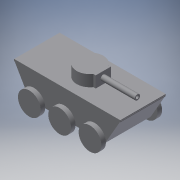
# Autodesk Inventor part: Part1
Saved by Autodesk Inventor 2019 (Build 230136000, 136)
## iProperties
Created: 2019-04-02
Part Number: Part1
Material: Generic
Document SubType Name: Modeling
Designer: Dainis-PC
Density: 1 g/cm^3
Appearance: Default
Author: Dainis-PC
Autodesk Inventor part; units mm, degrees
ref_plane "YZ Plane" through (0, 0, 0) normal (1, 0, 0) x (0, 1, 0)
ref_plane "XZ Plane" through (0, 0, 0) normal (0, 1, 0) x (-1, 0, 0)
ref_plane "XY Plane" through (0, 0, 0) normal (0, 0, 1) x (1, 0, 0)
sketch "Sketch1" plane through (0, 0, 0) normal (0, 0, 1) x (1, 0, 0)
  line L0 (0, 0) -> (200, 0)
  line L1 (0, 0) -> (-40, 69.282)
  line L2 (0, 0) -> (80, 0) construction
  line L3 (200, 0) -> (240, 69.282)
  line L4 (200, 0) -> (280, 0) construction
  line L5 (-40, 69.282) -> (240, 69.282)
  dimension "d0" = 200
  dimension "d1" = 80
  dimension "d2" = 120
  dimension "d3" = 80
  dimension "d4" = 60
  constraints: 12 end point, 3 horizontal, 2 equal length
  measures "d0" distance of L0.start L0.end
  measures "d1" distance of L0.start L1.end
  measures "d2" angle of L2 L1
  measures "d3" distance of L0.end L3.end
  measures "d4" angle of L4 L3
sketch "Sketch2" plane through (0, 0, 0) normal (0, 1, 0) x (-1, 0, 0)
  line L0 (0, 0) -> (0, -120)
  line L1 (0, -120) -> (-200, -120)
  line L2 (-200, -120) -> (-200, 0)
  dimension "d5" = 120
  dimension "d6" = 200
  constraints: 6 end point, 2 perpendicular, 1 vertical
  measures "d5" distance of L0.start L0.end
  measures "d6" distance of L0.end L1.end
extrude "Extrusion1" add sketch "Sketch1" against normal blind 5
extrude "Extrusion2" add sketch "Sketch2" along normal blind 5 fills toward (-0.05, -60) open curves L0 L1 L2
sketch "Sketch3" plane through (200, 0, -120) normal (0, 0, -1) x (-1, 0, 0)
  line L0 (200, 0) -> (0, 0) projected
  line L1 (-40, 69.282) -> (0, 0) projected
  line L2 (0, 0) -> (-40, 69.282)
  line L3 (240, 69.282) -> (-40, 69.282) projected
  line L4 (-40, 69.282) -> (240, 69.282)
  line L5 (240, 69.282) -> (200, 0)
  line L6 (0, 0) -> (200, 0)
  line L7 (0, 5) -> (200, 5) projected
  constraints: 8 end point, 3 equal length
extrude "Extrusion3" add sketch "Sketch3" against normal blind 5
sketch "Sketch4" plane through (240, 69.282, 0) normal (0.8660254, -0.5, 0) x (0, 0, -1)
  line L0 (0, 0) -> (5, 0) projected
  line L1 (0, 0) -> (120, 0)
  line L2 (120, -80) -> (115, -80) projected
  line L3 (120, 0) -> (120, -80)
  line L4 (120, -80) -> (0, -80)
  line L5 (5, -75.6699) -> (115, -75.6699) projected
  line L6 (0, -80) -> (0, 0)
  line L7 (5, 0) -> (5, -80) projected
  point P0 (0, -180)
  constraints: 8 end point, 2 parallel, 1 horizontal, 1 perpendicular
extrude "Extrusion4" add sketch "Sketch4" against normal blind 5 contours L1 L3 L2 L4 L7
sketch "Sketch5" plane through (0, 0, -120) normal (-0.8660254, -0.5, 0) x (0, 0, 1)
  line L0 (120, 0) -> (0, 0)
  line L1 (0, 0) -> (0, 80) projected
  line L2 (0, 0) -> (0, 80)
  line L3 (0, 80) -> (120, 80)
  line L4 (120, 80) -> (120, 0)
  constraints: 8 end point, 1 horizontal, 1 perpendicular
extrude "Extrusion5" add sketch "Sketch5" against normal blind 5
sketch "Sketch6" plane through (-34.2265, 69.282, -120) normal (0, 1, 0) x (1, 0, 0)
  line L0 (34.2265, 0) -> (-5.7735, 0) projected
  line L1 (-5.7735, 0) -> (-5.7735, -120)
  line L2 (-5.7735, -120) -> (274, -120)
  line L3 (-5.7735, -120) -> (34.2265, -120) projected
  line L4 (274, -120) -> (274, 0)
  line L5 (269.8964, -115) -> (269.8964, 0) projected
  line L6 (274, 0) -> (-5.7735, 0)
  line L7 (268.453, -5) -> (0, -5) projected
  constraints: 8 end point, 2 parallel, 1 collinear, 1 vertical
extrude "Extrusion6" add sketch "Sketch6" along normal mid plane 5
sketch "Sketch7" plane through (0, 0, 0) normal (0, 0, 1) x (1, 0, 0)
  line L0 (-38.5566, 66.782) -> (0, 0) projected
  circle A0 centre (20, 10) radius 4
  circle A1 centre (180, 10) radius 4
  circle A2 centre (100, 10) radius 4
  point P0 (200, 0)
  constraints: 3 centre point
extrude "Extrusion7" add sketch "Sketch7" along normal blind 8
sketch "Sketch8" plane through (20, 10, 8) normal (0, 0, 1) x (1, 0, 0)
  circle A0 centre (0, 0) radius 4 projected
  circle A1 centre (0, 0) radius 30
  circle A2 centre (80, 0) radius 4 projected
  circle A3 centre (80, 0) radius 30
  circle A4 centre (160, 0) radius 4 projected
  circle A5 centre (160, 0) radius 30
  point P0 (-20, -10)
  constraints: 3 centre point, 3 coincident
extrude "Extrusion8" add sketch "Sketch8" along normal blind 12 contours A0 | A1 | A2 | A3 | A4 | A5
sketch "Sketch9" plane through (200, 0, -120) normal (0, 0, -1) x (-1, 0, 0)
  circle A0 centre (180, 10) radius 4 projected
  circle A1 centre (180, 10) radius 4
  circle A2 centre (100, 10) radius 4 projected
  circle A3 centre (100, 10) radius 4
  circle A4 centre (20, 10) radius 4 projected
  circle A5 centre (20, 10) radius 4
  point P0 (200, 0)
  constraints: 3 centre point, 3 coincident
extrude "Extrusion9" add sketch "Sketch9" along normal blind 8
sketch "Sketch10" plane through (100, 10, -128) normal (0, 0, -1) x (-1, 0, 0)
  circle A0 centre (0, 0) radius 4 projected
  circle A1 centre (0, 0) radius 30
  circle A2 centre (80, 0) radius 30 projected
  circle A3 centre (80, 0) radius 30
  circle A4 centre (-80, 0) radius 4 projected
  circle A5 centre (-80, 0) radius 30
  point P0 (100, -10)
  dimension "d32" = 60
  constraints: 3 centre point, 3 coincident
  measures "d32" diameter of A1
extrude "Extrusion10" add sketch "Sketch10" along normal blind 12 contours A0 | A1 | A2 | A4 | A5
sketch "Sketch11" plane through (-34.2265, 71.782, -120) normal (0, 1, 0) x (1, 0, 0)
  circle A0 centre (134.2265, -60) radius 35
  point P0 (34.2265, -120)
  dimension "d36" = 70
  constraints: 1 centre point
  measures "d36" diameter of A0
extrude "Extrusion11" add sketch "Sketch11" along normal blind 30
sketch "Sketch12" plane through (-34.2265, 71.782, -120) normal (0, 1, 0) x (1, 0, 0)
  circle A0 centre (134.2265, -60) radius 35 projected
  line L0 (169.2265, -60) -> (169.2265, -40)
  line L1 (169.2265, -40) -> (159.2265, -40)
  line L2 (159.2265, -40) -> (159.2265, -80)
  line L3 (159.2265, -80) -> (169.2265, -80)
  line L4 (169.2265, -80) -> (169.2265, -60)
  point P0 (34.2265, -120)
  dimension "d39" = 20
  dimension "d40" = 10
  dimension "d41" = 40
  constraints: 10 end point, 4 perpendicular, 3 vertical, 1 horizontal alignment, 1 point on line, 1 other
  measures "d39" distance of L0.start L0.end
  measures "d40" distance of L0.end L1.end
  measures "d41" distance of L1.end L2.end
extrude "Extrusion12" add sketch "Sketch12" along normal blind 30 contours A0 L3 L2 L1 | L4 L3 A0 | A0 L1 L0 picked at (162.5598, -60)
sketch "Sketch13" plane through (135, 71.782, -40) normal (1, 0, 0) x (0, 0, -1)
  line L0 (55, 30) -> (-15, 30) projected
  circle A0 centre (20, 15) radius 7
  point P0 (-40, -71.782)
  point P1 (0, 30)
  point P2 (40, 30)
  constraints: 1 centre point
extrude "Extrusion13" add sketch "Sketch13" along normal blind 90
sketch "Sketch14" plane through (225, 86.782, -60) normal (1, 0, 0) x (0, 0, -1)
  circle A0 centre (0, 0) radius 4
  point P0 (-60, -86.782)
  constraints: 1 centre point
extrude "Extrusion14" cut sketch "Sketch14" against normal blind 90
body "Solid1"
